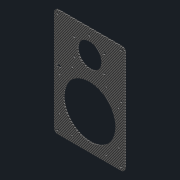
# Autodesk Inventor part: carbonplate3
Saved by Autodesk Inventor 2022 (Build 260153000, 153)
## iProperties
Created: 2021-09-16
Part Number: carbonplate3
Material: CFRP
Document SubType Name: Sheet Metal
Designer: Yuta Kage
Density: 1.43 g/cm^3
Sheet Metal Rule: Default_mm
Appearance: カーボンファイバー
Author: Yuta Kage
Autodesk Inventor part; units mm, degrees
ref_plane "YZ Plane" through (0, 0, 0) normal (1, 0, 0) x (0, 1, 0)
ref_plane "XZ Plane" through (0, 0, 0) normal (0, 1, 0) x (-1, 0, 0)
ref_plane "XY Plane" through (0, 0, 0) normal (0, 0, 1) x (1, 0, 0)
sketch "スケッチ1" plane through (0, 0, 0) normal (0, 0, 1) x (1, 0, 0)
  line L0 (55, -93.4) -> (-55, -93.4)
  line L1 (-55, -93.4) -> (-55, 75)
  line L2 (-55, 75) -> (55, 75)
  line L3 (55, 75) -> (55, -93.4)
  line L4 (55, -93.4) -> (-55, 75) construction
  line L5 (-55, -93.4) -> (55, 75) construction
  point P0 (0, 0)
  point P1 (0, -9.2)
  point P2 (0, -9.2)
  dimension "d50" = 93.4
  dimension "d51" = 110
  dimension "d52" = 75
  measures "d50" distance from line of L0 point (0, 0)
  measures "d51" distance of L0.start L0.end
  measures "d52" distance from line of point (0, 0) L2
extrude "プレート1" add sketch "スケッチ1" along normal blind 2
sketch "スケッチ3" plane through (0, 0, 2) normal (0, 0, 1) x (1, 0, 0)
  circle A0 centre (0, 38.4) radius 19
  circle A1 centre (0, -38.4) radius 10
  point P0 (0, 0)
  dimension "d22" = 38
  dimension "d53" = 20
  dimension "d55" = 76.8
  dimension "d56" = 38.4
  constraints: 2 centre point, 2 vertical alignment
  measures "d22" diameter of A0
  measures "d53" diameter of A1
  measures "d55" distance of A0.centre A1.centre
  measures "d56" distance of point (0, 0) A1.centre
extrude "押し出し1" cut sketch "スケッチ3" against normal blind 10 contours A0
sketch "スケッチ2" plane through (0, 0, 2) normal (0, 0, 1) x (1, 0, 0)
  circle A0 centre (0, 38.4) radius 15 construction
  circle A1 centre (0, -38.4) radius 53.5
  point P0 (0, 0)
  point P1 (0, 53.4)
  point P2 (-15, 38.4)
  point P3 (0, 23.4)
  point P4 (15, 38.4)
  point P5 (-46.3324, -11.65)
  point P6 (-53.5, -38.4)
  point P7 (-46.3324, -65.15)
  point P8 (-26.75, -84.7324)
  point P9 (0, -91.9)
  point P10 (26.75, -84.7324)
  point P11 (46.3324, -65.15)
  point P12 (53.5, -38.4)
  point P13 (46.3324, -11.65)
  point P14 (26.75, 7.9324)
  point P15 (0, 15.1)
  point P16 (-26.75, 7.9324)
  dimension "d3" = 30
  dimension "d8" = 107
  dimension "d6" = 360
  dimension "d11" = 360
  dimension "d13" = 76.8
  dimension "d14" = 38.4
  dimension "d58" = 0
  constraints: 3 vertical alignment, 2 horizontal alignment, 23 other
  measures "d13" distance of point (0, 38.4) point (0, -38.4)
  measures "d14" distance of point (0, 0) point (0, 38.4)
  measures "d58" horizontal distance of point (0, -38.4) point (0, -91.9)
hole "穴1" at (-26.75, -84.7324, 2) at (-46.3324, -65.15, 2) at (-26.75, 7.9324, 2) at (-46.3324, -11.65, 2) at (26.75, 7.9324, 2) at (46.3324, -11.65, 2) at (46.3324, -65.15, 2) at (26.75, -84.7324, 2) direction (0, 0, -1) diameter 3.2 end through all clearance for "Socket Head Cap Screw" size "M3" standard "Ansi Metric M Profile"
sketch "スケッチ4" plane through (0, 0, 2) normal (0, 0, 1) x (1, 0, 0)
  line L0 (55, -93.4) -> (-55, -93.4) projected
  line L1 (-55, -93.4) -> (-55, 75) projected
  line L2 (55, 75) -> (55, -93.4) projected
  line L3 (-55, 75) -> (55, 75) projected
  line L4 (-50, 70) -> (-50, -88.4)
  line L5 (-50, -88.4) -> (50, -88.4)
  line L6 (50, -88.4) -> (50, 70)
  line L7 (50, 70) -> (-50, 70)
  point P0 (-50, 0)
  point P1 (50, 0)
  point P2 (0, 0)
  dimension "d57" = 5
  constraints: 8 end point, 2 horizontal alignment, 2 point on line, 3 other
  measures "d57" distance between parallel lines of L1 L4
hole "穴2" at (-50, -88.4, 2) at (50, -88.4, 2) at (50, 70, 2) at (-50, 70, 2) at (-50, 0, 2) at (50, 0, 2) direction (0, 0, -1) diameter 4.3 end through all clearance for "Socket Head Cap Screw" size "M4" standard "Ansi Metric M Profile"
fillet "コーナーR1" radius 5 4 edges at (-55, -93.4, 1) (55, -93.4, 1) (55, 75, 1) (-55, 75, 1)
sketch "スケッチ5" plane through (0, 0, 2) normal (0, 0, 1) x (1, 0, 0)
  circle A0 centre (0, -38.4) radius 41
  point P0 (0, 0)
  dimension "d35" = 82
  constraints: 1 centre point, 1 coincident
  measures "d35" diameter of A0
extrude "押し出し2" cut sketch "スケッチ5" against normal blind 10
sketch "スケッチ6" plane through (0, 0, 2) normal (0, 0, 1) x (1, 0, 0)
  circle A0 centre (0, 38.4) radius 19 projected
  circle A1 centre (0, 38.4) radius 27
  point P0 (0, 0)
  point P1 (-23.3827, 51.9)
  point P2 (-23.3827, 24.9)
  point P3 (0, 11.4)
  point P4 (23.3827, 24.9)
  point P5 (23.3827, 51.9)
  point P6 (0, 65.4)
  dimension "d38" = 54
  dimension "d41" = 360
  dimension "d59" = 0
  constraints: 1 coincident, 10 other
  measures "d59" horizontal distance of point (23.383, 51.9) point (23.383, 24.9)
hole "穴3" at (0, 65.4, 2) at (23.3827, 51.9, 2) at (23.3827, 24.9, 2) at (-23.3827, 24.9, 2) at (-23.3827, 51.9, 2) direction (0, 0, -1) diameter 4.3 end through all clearance for "Socket Head Cap Screw" size "M4" standard "Ansi Metric M Profile"
sketch "スケッチ7" plane through (0, 0, 2) normal (0, 0, 1) x (1, 0, 0)
  circle A0 centre (-50, 0) radius 2.15 projected
  line L0 (-46.2, 0) -> (-50, 0) construction
  line L1 (-46.2, 2.15) -> (-50, 2.15)
  line L2 (-50, -2.15) -> (-46.2, -2.15)
  arc A1 (-46.2, -2.15) -> (-46.2, 2.15) centre (-46.2, 0) ccw
  arc A2 (-50, 2.15) -> (-50, -2.15) centre (-50, 0) ccw
  point P0 (0, 0)
  point P1 (-48.1, 0)
  dimension "d60" = 48.1
  constraints: 8 end point, 5 tangent, 4 point on circle, 2 centre point, 1 horizontal, 1 midpoint, 1 parallel
  measures "d60" distance of point (0, 0) point (-48.1, 0)
extrude "押し出し3" cut sketch "スケッチ7" against normal through all
equation "\"d56\" = 0.5 * d55"
equation "\"d14\" = 0.5 * d13"
equation "\"d20\" = Thickness"
equation "\"d2\" = Thickness"
equation "\"BendRadius\" = Thickness"
equation "\"BendReliefWidth\" = Thickness"
equation "\"BendReliefDepth\" = 0.5 * Thickness"
equation "\"CornerReliefSize\" = 4 * Thickness"
equation "\"MinimumRemnant\" = 2 * Thickness"
equation "\"TransitionRadius\" = BendRadius"
equation "\"JacobiRadiusSize\" = BendRadius"
equation "\"GapSize\" = Thickness"
equation "\"Thickness\" = 2"
